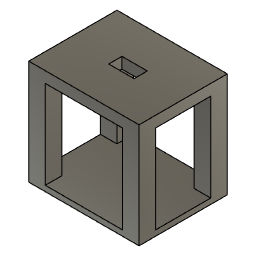
Postolje stacionarni (Autodesk Fusion 360 design; units mm, degrees)
Autodesk Fusion 360 part; units mm, degrees
note: some values were not read from the file. Set by a fixed rule: which sketch regions a step uses.
sketch "Sketch3" plane through (0, 0, 0) normal (0, 0, 1) x (1, 0, 0)
  line L0 (50, -40) -> (-50, -40)
  line L1 (-50, -40) -> (-50, 40)
  line L2 (-50, 40) -> (50, 40)
  line L3 (50, 40) -> (50, -40)
  line L4 (50, -40) -> (-50, 40) construction
  line L5 (-50, -40) -> (50, 40) construction
  line L6 (35, -26.5) -> (-35, -26.5)
  line L7 (-35, -26.5) -> (-35, 26.5)
  line L8 (-35, 26.5) -> (35, 26.5)
  line L9 (35, 26.5) -> (35, -26.5)
  line L10 (35, -26.5) -> (-35, 26.5) construction
  line L11 (-35, -26.5) -> (35, 26.5) construction
  line L12 (-50, 40) -> (-35, 40)
  line L13 (-35, 40) -> (-35, 25)
  line L14 (-35, 25) -> (-50, 25)
  line L15 (-50, 25) -> (-50, 40)
  line L16 (50, 40) -> (35, 40)
  line L17 (35, 40) -> (35, 25)
  line L18 (35, 25) -> (50, 25)
  line L19 (50, 25) -> (50, 40)
  line L20 (50, -40) -> (35, -40)
  line L21 (35, -40) -> (35, -25)
  line L22 (35, -25) -> (50, -25)
  line L23 (50, -25) -> (50, -40)
  line L24 (-50, -40) -> (-35, -40)
  line L25 (-35, -40) -> (-35, -25)
  line L26 (-35, -25) -> (-50, -25)
  line L27 (-50, -25) -> (-50, -40)
  dimension "d8" = 100
  dimension "d9" = 80
  dimension "d10" = 70
  dimension "d11" = 53
  dimension "d19" = 15
  dimension "d20" = 15
  dimension "d21" = 15
  dimension "d22" = 15
  dimension "d23" = 15
  dimension "d24" = 15
  dimension "d25" = 15
  dimension "d26" = 15
  constraint horizontal L0
  constraint perpendicular L0 L1
  constraint parallel L0 L2
  constraint parallel L1 L3
  constraint coincident L4 origin
  constraint coincident L5 origin
  constraint horizontal L6
  constraint perpendicular L6 L7
  constraint parallel L6 L8
  constraint parallel L7 L9
  constraint coincident L10 origin
  constraint coincident L11 origin
  constraint horizontal L12
  constraint vertical L13
  constraint horizontal L14
  constraint vertical L15
  constraint horizontal L16
  constraint vertical L17
  constraint horizontal L18
  constraint vertical L19
  constraint horizontal L20
  constraint vertical L21
  constraint horizontal L22
  constraint vertical L23
  constraint horizontal L24
  constraint vertical L25
  constraint horizontal L26
  constraint vertical L27
  measures "d8" distance of L1.end L2.end
  measures "d9" distance of L0.end L1.end
  measures "d10" distance of L7.end L8.end
  measures "d11" distance of L6.end L7.end
  measures "d19" distance of L12.end L13.end
  measures "d20" distance of L13.end L14.end
  measures "d21" distance of L16.end L17.end
  measures "d22" distance of L17.end L18.end
  measures "d23" distance of L21.end L22.end
  measures "d24" distance of L20.end L21.end
  measures "d25" distance of L25.end L26.end
  measures "d26" distance of L24.end L25.end
extrude "Extrude3" add sketch "Sketch3" along normal blind 80 contours L0 L3 L9 L20 L21 L22 L23 | L0 L1 L7 L24 L25 L26 L27 | L2 L3 L9 L16 L17 L18 L19 | L1 L2 L7 L12 L13 L14 L15 makes body 1 at (40, 25, 26.6667) makes body 2 at (45, -40, 26.6667) makes body 3 at (-50, 30, 26.6667) makes body 4 at (-40, -40, 26.6667)
extrude "Extrude4" add sketch "Sketch3" against normal blind 5 bodies 1 2 3 4
ref_plane "WorkPlane2" through (-42.5, 32.5, 80) normal (0, 0, 1) x (1, 0, 0)
sketch "Sketch4" plane through (-40, 30, 80) normal (0, 0, 1) x (1, 0, 0)
  line L0 (-10, 10) -> (90, 10)
  line L1 (90, 10) -> (90, -70)
  line L2 (90, -70) -> (-10, -70)
  line L3 (-10, -70) -> (-10, 10)
  constraint horizontal L0
  constraint vertical L1
  constraint horizontal L2
  constraint vertical L3
extrude "Extrude5" add sketch "Sketch4" along normal blind 10 bodies 1
sketch "Sketch5" plane through (0, 0, 90) normal (0, 0, 1) x (-1, 0, 0)
  line L0 (50, 40) -> (-50, 40)
  line L1 (-50, 40) -> (-50, -40)
  line L2 (-50, -40) -> (50, -40)
  line L3 (50, -40) -> (50, 40)
  line L4 (-11.5, 6) -> (11.5, 6)
  line L5 (11.5, 6) -> (11.5, -6)
  line L6 (11.5, -6) -> (-11.5, -6)
  line L7 (-11.5, -6) -> (-11.5, 6)
  line L8 (-11.5, 6) -> (11.5, -6) construction
  line L9 (11.5, 6) -> (-11.5, -6) construction
  dimension "d27" = 23
  dimension "d28" = 12
  constraint horizontal L4
  constraint perpendicular L4 L5
  constraint parallel L4 L6
  constraint parallel L5 L7
  constraint coincident L8 origin
  constraint coincident L9 origin
  measures "d27" distance of L5.end L6.end
  measures "d28" distance of L4.end L5.end
extrude "Extrude6" cut sketch "Sketch5" against normal blind 15 contours L4 L5 L6 L7 bodies 1
